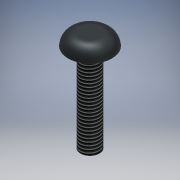
# Autodesk Inventor part: M3トラス頭ネジ　14
Saved by Autodesk Inventor 2017.3 (Build 213256000, 256)
## iProperties
Part Number: M3トラス頭ネジ　14
Material: 鉄 灰色
Document SubType Name: Modeling
Designer: 原知也
Density: 7.15 g/cm^3
Appearance: 鉄 灰色
Author: 原知也
Autodesk Inventor part; units mm, degrees
ref_plane "YZ Plane" through (0, 0, 0) normal (1, 0, 0) x (0, 1, 0)
ref_plane "XZ Plane" through (0, 0, 0) normal (0, 1, 0) x (-1, 0, 0)
ref_plane "XY Plane" through (0, 0, 0) normal (0, 0, 1) x (1, 0, 0)
sketch "スケッチ1" plane through (0, 0, 0) normal (0, 0, 1) x (1, 0, 0)
  circle A0 centre (0, 0) radius 1.5
  dimension "d0" = 3
  constraints: 1 centre point, 1 coincident
  measures "d0" diameter of A0
extrude "押し出し1" add sketch "スケッチ1" along normal blind 14
sketch "スケッチ2" plane through (0, 0, 14) normal (0, 0, 1) x (1, 0, 0)
  circle A0 centre (0, 0) radius 3.45
  dimension "d3" = 6.9
  constraints: 1 centre point, 1 coincident
  measures "d3" diameter of A0
extrude "押し出し2" add sketch "スケッチ2" along normal blind 1.9
fillet "フィレット1" radius 1.9 1 edges at (-3.45, 0, 15.9)
thread "ねじ1" size "M3x0.5" class "6g" standard "ANSI Metric M Profile" full length
